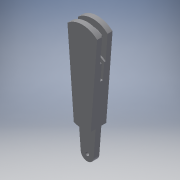
# Autodesk Inventor part: poker
Saved by Autodesk Inventor 2018 (Build 220112000, 112)
## iProperties
Created: 2017-12-11
Part Number: poker
Material: Generic
Document SubType Name: Modeling
Designer: ragna
Density: 1 g/cm^3
Appearance: Default
Author: ragna
Autodesk Inventor part; units mm, degrees
ref_plane "YZ Plane" through (0, 0, 0) normal (1, 0, 0) x (0, 1, 0)
ref_plane "XZ Plane" through (0, 0, 0) normal (0, 1, 0) x (-1, 0, 0)
sketch "Sketch1" plane through (0, 0, 0) normal (0, 0, 1) x (1, 0, 0)
  arc A0 (-0.1713, -0.9133) -> (-5.7787, -0.9133) centre (-2.975, -4.7604) ccw
  arc A1 (-5.7787, -1.5867) -> (-0.1713, -1.5867) centre (-2.975, 2.2604) ccw
  circle A2 centre (-5.5333, -1.25) radius 0.4167
  circle A3 centre (-0.4167, -1.25) radius 0.4167
  line L0 (-5.95, 0) -> (0, 0)
  line L1 (0, 0) -> (0, -2.5)
  line L2 (0, -2.5) -> (-5.95, -2.5)
  line L3 (-5.95, -2.5) -> (-5.95, 0)
  point P0 (-1.5, -3.25)
  dimension "d8" = 4.7604
  dimension "d11" = 0.8333
  dimension "d12" = 5.95
  dimension "d13" = 2.5
  dimension "d14" = 0.8333
  dimension "d22" = 4.7604
  constraints: 8 end point, 8 point on circle, 8 tangent, 4 centre point, 2 parallel, 1 coincident, 1 horizontal, 1 perpendicular, 1 vertical alignment
  measures "d8" radius of A0
  measures "d11" diameter of A3
  measures "d12" distance of L1.end L2.end
  measures "d13" distance of L2.end L0.start
  measures "d14" diameter of A2
  measures "d22" radius of A1
extrude "Extrusion1" add sketch "Sketch1" against normal blind 0.6 contours A3 A1 A2 A0 | A3 | A2
sketch "Sketch2" plane through (0, 0, 0) normal (0, 0, 1) x (1, 0, 0)
  arc A0 (-0.1713, -0.9133) -> (-5.7787, -0.9133) centre (-2.975, -4.7604) ccw projected
  arc A1 (1.575, 0.2396) -> (-7.525, 0.2396) centre (-2.975, -4.7604) ccw
  line L0 (-4.9692, -33.1526) -> (-7.525, 0.2396)
  line L1 (-0.9808, -33.1526) -> (1.575, 0.2396)
  circle A2 centre (-2.975, -33) radius 2
  arc A3 (-0.1713, -0.9133) -> (-5.7787, -0.9133) centre (-2.975, -4.7604) ccw projected
  line L2 (-11.9492, 2) -> (-1.5879, 2) construction
  point P0 (-7.5, -3.25)
  dimension "d15" = 33.4899
  dimension "d16" = 2
  dimension "d17" = 33.4899
  dimension "d19" = 4
  dimension "d20" = 9.1
  dimension "d21" = 35
  constraints: 6 end point, 4 point on circle, 3 tangent, 2 centre point, 1 horizontal, 1 vertical alignment, 1 other
  measures "d15" distance of L0.start L0.end
  measures "d17" distance of L1.start L1.end
  measures "d19" diameter of A2
  measures "d20" distance of L1.end L0.end
  measures "d21" distance from line of L2 A2.centre
extrude "Extrusion2" add sketch "Sketch2" along normal blind 1.5
sketch "Sketch4" plane through (0, 0, 0) normal (0, 0, -1) x (-1, 0, 0)
  arc A0 (7.525, 0.2396) -> (-1.575, 0.2396) centre (2.975, -4.7604) ccw projected
  line L0 (4.6338, -2.5) -> (0.9036, -2.5) construction
  line L1 (4.4698, -6) -> (1.0404, -6) construction
  arc A1 (0.1713, -1.5867) -> (5.7787, -1.5867) centre (2.975, 2.2604) ccw construction
  line L2 (7.525, 0.2396) -> (4.9692, -33.1526) construction
  line L3 (0.9808, -33.1526) -> (-1.575, 0.2396) construction
  arc A2 (6.9486, -7.2911) -> (-0.9986, -7.2911) centre (2.975, -12.7604) ccw
  line L4 (7.525, 0.2396) -> (4.9692, -33.1526) construction
  line L5 (0.9808, -33.1526) -> (-1.575, 0.2396) construction
  arc A3 (0.9808, -33.1526) -> (4.9692, -33.1526) centre (2.975, -33) ccw projected
  line L6 (6.9486, -7.2911) -> (4.9692, -33.1526)
  line L7 (0.9808, -33.1526) -> (-0.9986, -7.2911)
  point P0 (0, 0)
  dimension "d23" = 3.5
  dimension "d24" = 6.7604
  dimension "d25" = 6.7604
  constraints: 8 end point, 3 point on circle, 3 tangent, 2 collinear, 2 horizontal, 2 point on line, 1 centre point, 1 horizontal alignment
  measures "d23" distance between parallel lines of L0 L1
  measures "d24" radius of A2
  measures "d25" radius of A0
extrude "Extrusion4" add sketch "Sketch4" along normal blind 0.85
sketch "Sketch7" plane through (0, 0, -0.85) normal (0, 0, -1) x (-1, 0, 0)
  arc A0 (6.9486, -7.2911) -> (-0.9986, -7.2911) centre (2.975, -12.7604) ccw projected
  line L0 (-0.9986, -7.2911) -> (0.9808, -33.1526) projected
  arc A1 (0.9808, -33.1526) -> (4.9692, -33.1526) centre (2.975, -33) ccw projected
  line L1 (4.9692, -33.1526) -> (6.9486, -7.2911) projected
  line L2 (-0.6188, -12.2527) -> (6.5688, -12.2527)
  point P0 (0, 0)
  constraints: 2 end point, 2 point on line, 1 horizontal
extrude "Extrusion7" cut sketch "Sketch7" against normal blind 0.4 contours L1 L2 L0 A0
sketch "Sketch3" plane through (0, 0, 1.5) normal (0, 0, 1) x (1, 0, 0)
  arc A0 (-4.9692, -33.1526) -> (-0.9808, -33.1526) centre (-2.975, -33) ccw projected
  circle A1 centre (-2.975, -33) radius 0.55
  point P0 (0, 0)
  dimension "d5" = 1.1
  constraints: 1 centre point, 1 coincident
  measures "d5" diameter of A1
extrude "Extrusion3" cut sketch "Sketch3" against normal through all
ref_plane "Work Plane1" through (-4.9692, -33.1526, -0.85) normal (0, 0, -1) x (-1, 0, 0)
mirror "Mirror1" about plane through (-2.975, -19.8303, -0.85) normal (0, 0, -1) of "Extrusion1", "Extrusion2", "Extrusion4", "Extrusion3", "Extrusion7"
sketch "Sketch8" plane through (-2.975, -4.7604, -3.2) normal (0, 0, -1) x (-1, 0, 0)
  circle A0 centre (0, -28.2396) radius 0.55 projected
  arc A1 (-1.9942, -28.3923) -> (1.9942, -28.3923) centre (0, -28.2396) ccw projected
  line L0 (4.55, 5) -> (1.9942, -28.3923) projected
  arc A2 (4.55, 5) -> (-4.55, 5) centre (0, 0) ccw projected
  line L1 (-1.9942, -28.3923) -> (-4.55, 5) projected
  line L2 (-1.9942, -28.3923) -> (-4.55, 5) projected
  line L3 (4.55, 5) -> (1.9942, -28.3923) projected
  arc A3 (-2.6101, -20.3444) -> (2.6101, -20.3444) centre (0, -14.1082) ccw
  point P0 (-2.975, 4.7604)
  dimension "d37" = 6.7604
  dimension "d38" = 6.7604
  constraints: 2 point on circle, 2 point on line, 1 centre point, 1 horizontal alignment
  measures "d37" radius of A3
  measures "d38" radius of A2
extrude "Extrusion8" cut sketch "Sketch8" against normal blind 1.5 contours L1 A3 L0 A1
mirror "Mirror2" about plane through (-4.9692, -33.1526, -0.85) normal (0, 0, -1) of "Extrusion8"
fillet "Fillet1" radius 0.2 8 edges at (-2.975, 0, -0.6) (0, -1.25, -0.6) (-2.975, -2.5, -0.6) (-5.95, -1.25, -0.6) (-2.975, 0, -1.1) (0, -1.25, -1.1) (-2.975, -2.5, -1.1) (-5.95, -1.25, -1.1)
sketch "Sketch6" plane through (-2.975, -4.7604, -3.2) normal (0, 0, -1) x (-1, 0, 0)
  line L0 (-1.9942, -28.3923) -> (-4.55, 5) projected
  line L1 (4.55, 5) -> (1.9942, -28.3923) projected
  arc A0 (-2.5344, -21.3343) -> (2.5344, -21.3343) centre (0, -18.2396) ccw
  circle A1 centre (0, -28.2396) radius 0.55 projected
  arc A2 (-1.9942, -28.3923) -> (1.9942, -28.3923) centre (0, -28.2396) ccw projected
  point P0 (-2.975, 4.7604)
  dimension "d31" = 4
  dimension "d32" = 10
  constraints: 2 point on circle, 2 point on line, 1 centre point, 1 horizontal alignment
  measures "d31" radius of A0
  measures "d32" distance of A1.centre A0.centre
equation "\"d11\" = 0.333333 * d13"
equation "\"d12\" = phheight"
equation "\"d13\" = phwidth"
equation "\"d14\" = d11"
equation "\"d22\" = d8"
equation "\"d16\" = phtosolid"
equation "\"d17\" = d15"
equation "\"d20\" = pheight"
equation "\"d24\" = d25"
equation "\"d37\" = d38"
equation "\"phtofree\" = 2.5"
equation "\"phtosolid\" = 2"
equation "\"phheight\" = 5.95"
equation "\"phwidth\" = 2.5"
equation "\"pheight\" = 9.1"
body "Solid1"
